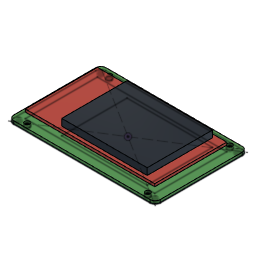
Brewi Gerät v7 (Autodesk Fusion 360 design; units mm, degrees)
Autodesk Fusion 360 part; units mm, degrees
sketch "Sketch1" plane through (0, 0, 0) normal (0, 1, 0) x (1, 0, 0)
  line L0 (40.7, -27.475) -> (-40.7, -27.475)
  line L1 (-43.7, -24.475) -> (-43.7, 24.475)
  line L2 (-40.7, 27.475) -> (40.7, 27.475)
  line L3 (43.7, 24.475) -> (43.7, -24.475)
  line L4 (43.7, -27.475) -> (-43.7, 27.475) construction
  line L5 (-43.7, -27.475) -> (43.7, 27.475) construction
  line L6 (-39.95, 21.675) -> (37.26, 21.675)
  line L7 (37.26, 21.675) -> (37.26, -21.325)
  line L8 (37.26, -21.325) -> (-39.95, -21.325)
  line L9 (-39.95, -21.325) -> (-39.95, 21.675)
  line L10 (-20.24, 19.675) -> (30.76, 19.675)
  line L11 (30.76, 19.675) -> (30.76, -19.325)
  line L12 (30.76, -19.325) -> (-20.24, -19.325)
  line L13 (-20.24, -19.325) -> (-20.24, 19.675)
  arc A0 (-40.7, 27.475) -> (-43.7, 24.475) centre (-40.7, 24.475) ccw
  arc A1 (43.7, 24.475) -> (40.7, 27.475) centre (40.7, 24.475) ccw
  arc A2 (40.7, -27.475) -> (43.7, -24.475) centre (40.7, -24.475) ccw
  arc A3 (-43.7, -24.475) -> (-40.7, -27.475) centre (-40.7, -24.475) ccw
  circle A4 centre (-35.7, 24.475) radius 1.5
  circle A5 centre (-35.7, -24.475) radius 1.5
  circle A6 centre (36.3, -24.475) radius 1.5
  circle A7 centre (36.3, 24.475) radius 1.5
  dimension "d1" = 87.4
  dimension "d2" = 54.95
  dimension "d3" = 77.21
  dimension "d4" = 43
  dimension "d5" = 6.44
  dimension "d6" = 5.8
  dimension "d7" = 51
  dimension "d8" = 39
  dimension "d9" = 6.5
  dimension "d10" = 2
  dimension "d17" = 3
  dimension "d18" = 3
  dimension "d19" = 3
  dimension "d20" = 3
  dimension "d21" = 3
  dimension "d22" = 8
  dimension "d23" = 3
  dimension "d24" = 3
  dimension "d25" = 3
  dimension "d26" = 8
  dimension "d27" = 3
  dimension "d29" = 3
  dimension "d30" = 3
  dimension "d31" = 3
  dimension "d33" = 72
  dimension "d34" = 72
  constraint horizontal L0
  constraint perpendicular L0 L1
  constraint parallel L0 L2
  constraint parallel L1 L3
  constraint coincident L4 origin
  constraint coincident L5 origin
  constraint horizontal L6
  constraint vertical L7
  constraint horizontal L8
  constraint vertical L9
  constraint horizontal L10
  constraint vertical L11
  constraint horizontal L12
  constraint vertical L13
  constraint coincident L4.end L1
  constraint coincident L4.end L2
  constraint tangent L1 A0
  constraint tangent L2 A0
  constraint coincident L5.end L2
  constraint coincident L5.end L3
  constraint tangent L2 A1
  constraint tangent L3 A1
  constraint coincident L4.start L3
  constraint coincident L4.start L0
  constraint tangent L3 A2
  constraint tangent L0 A2
  constraint coincident L5.start L0
  constraint coincident L5.start L1
  constraint tangent L0 A3
  constraint tangent L1 A3
  measures "d1" distance of L4.end L5.end
  measures "d2" distance of L5.start L4.end
  measures "d3" distance of L6.start L6.end
  measures "d4" distance of L6.start L8.end
  measures "d5" distance of L3 L7
  measures "d6" distance of L2 L6
  measures "d7" distance of L10.start L10.end
  measures "d8" distance of L10.start L12.end
  measures "d9" distance of L7 L11
  measures "d10" distance of L6 L10
  measures "d17" radius of A0
  measures "d18" radius of A1
  measures "d19" radius of A2
  measures "d20" radius of A3
  measures "d21" diameter of A4
  measures "d22" distance of L1 A4.centre
  measures "d23" distance of L2 A4.centre
  measures "d24" diameter of A5
  measures "d25" distance of L0 A5.centre
  measures "d26" distance of L1 A5.centre
  measures "d27" diameter of A6
  measures "d29" distance of L0 A6.centre
  measures "d30" diameter of A7
  measures "d31" distance of L2 A7.centre
  measures "d33" distance of A4.centre A7.centre
  measures "d34" distance of A5.centre A6.centre
extrude "Extrude1" add sketch "Sketch1" along normal blind 4 contours L10 L11 L12 L13 makes body 1
extrude "Extrude2" add sketch "Sketch1" 1 faces at (-3.24, 0, 6.325) against normal blind 1.6 separate body contours L6 L7 L8 L9 | L10 L11 L12 L13 on bodies 1 makes body 2
move_body "Move1" bodies 2 1 to x (1, 0, 0) y (0, 1, 0) z (0, 0, 1) at (0, 5, 0)
extrude "Extrude3" add sketch "Sketch1" along normal blind 1.6 separate body contours L0 L1 L2 L3 A0 A1 A2 A3 | L6 L7 L8 L9 | L10 L11 L12 L13 makes body 3
named bodies: "Display", "Rote Platine", "Grüne Platine"
